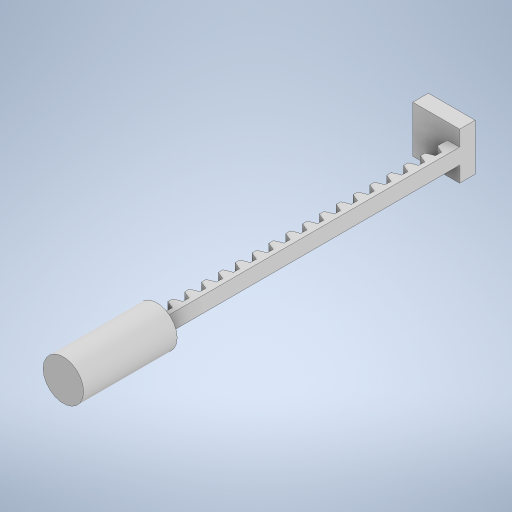
# Autodesk Inventor part: Lineartranslator
Saved by Autodesk Inventor 2024 (Build 280153000, 153)
## iProperties
Created: 2024-01-09
Part Number: Lineartranslator
Material: Generisch
Document SubType Name: Modeling
Designer: mariu
Density: 1 g/cm^3
Appearance: Vorgabe
Author: mariu
Autodesk Inventor part; units mm, degrees
ref_plane "YZ Plane" through (0, 0, 0) normal (1, 0, 0) x (0, 1, 0)
ref_plane "XZ Plane" through (0, 0, 0) normal (0, 1, 0) x (-1, 0, 0)
ref_plane "XY Plane" through (0, 0, 0) normal (0, 0, 1) x (1, 0, 0)
sketch "Skizze2" plane through (0, 0, 0) normal (0, 0, 1) x (1, 0, 0)
  circle A0 centre (0, 0) radius 12.5 construction
  circle A1 centre (0, 0) radius 15
  line L0 (-15, 0) -> (-12.5, 0)
  arc A2 (-12.4599, -1) -> (-14.8661, -2) centre (-8.8919, -12.9799) ccw
  arc A3 (-14.8661, 2) -> (-12.4599, 1) centre (-8.8919, 12.9799) ccw
  arc A4 (-14.8661, 2) -> (-14.8661, -2) centre (0, 0) ccw
  arc A5 (-12.4599, 1) -> (-12.4599, -1) centre (0, 0) ccw
  circle A6 centre (0, 0) radius 15
  line L1 (-12.4599, 1) -> (-12.4599, -1)
  line L2 (-12.4599, 1) -> (-12.4599, 21)
  line L3 (-12.4599, -1) -> (-12.4599, -21)
  line L4 (-14.8661, -2) -> (-14.8661, -21)
  line L5 (-12.4599, -21) -> (-14.8661, -21)
  line L6 (-14.8661, 2) -> (-14.8661, 21)
  line L7 (-14.8661, 21) -> (-12.4599, 21)
  line L8 (-12.4599, 21) -> (-10.9599, 21)
  line L9 (-10.9599, 21) -> (-10.9599, -21)
  line L10 (-10.9599, -21) -> (-12.4599, -21)
  line L11 (-14.8661, 2) -> (-14.8661, 2.9)
  line L12 (-14.8661, 2.9) -> (-12.4599, 2.9)
  line L13 (-14.8661, -2) -> (-14.8661, -2.9)
  line L14 (-14.8661, -2.9) -> (-12.4599, -2.9)
  point P0 (-13.75, 0)
  point P1 (-15, 0)
  point P2 (-12.4599, -8.3516)
  point P3 (-10.9599, -10.2411)
  point P4 (-10.9599, 10.2411)
  point P5 (-12.4599, 8.3516)
  dimension "d5" = 25
  dimension "d6" = 12.5
  dimension "d7" = 4
  dimension "d8" = 2
  dimension "d9" = 13.75
  dimension "d11" = 30
  dimension "d12" = 20
  dimension "d13" = 20
  dimension "d14" = 1.5
  dimension "d17" = 0.9
  dimension "d18" = 0.9
  constraints: 30 end point, 15 point on circle, 7 centre point, 7 coincident, 6 perpendicular, 6 point on line, 3 horizontal, 2 concentric, 2 vertical, 1 horizontal alignment, 1 midpoint, 1 other
  measures "d5" diameter of A0
  measures "d6" radius of A2
  measures "d7" distance of L6.start L4.start
  measures "d8" distance of L1.start L1.end
  measures "d9" distance of point (0, 0) point (-13.75, 0)
  measures "d11" diameter of A6
  measures "d12" distance of L1.start L2.end
  measures "d13" distance of L1.end L3.end
  measures "d14" distance of L2.end L8.end
  measures "d17" distance of L6.start L11.end
  measures "d18" distance of L4.start L13.end
extrude "Extrusion1" add sketch "Skizze2" along normal blind 5 contours L6 L12 A1 | A1 L12 L2 A3 | L2 A1 L9 L3 L1 | A2 L3 L14 A1 | A1 L14 L4
pattern_linear "Rechteckige Anordnung1" count 20 spacing 5.4 along (0, 1, 0) of "Extrusion1"
sketch "Skizze3" plane through (-12.4599, 105.5, 0) normal (-1, 0, 0) x (0, 0, 1)
  line L0 (5, -115.7411) -> (5, 7.3411) projected
  line L1 (5, 2.3411) -> (0, 2.3411)
  line L2 (0, -115.7411) -> (0, 7.3411) projected
  line L3 (0, 2.3411) -> (0, 7.3411)
  line L4 (0, 7.3411) -> (5, 7.3411)
  line L5 (5, 7.3411) -> (5, 2.3411)
  point P0 (0, -105.5)
  point P1 (2.5, 7.3411)
  dimension "d22" = 5
  constraints: 8 end point, 3 perpendicular, 1 horizontal, 1 midpoint, 1 point on line
  measures "d22" distance from line of point (2.5, 7.341) L1
extrude "Extrusion2" cut sketch "Skizze3" against normal blind 5
sketch "Skizze4" plane through (-12.4599, 107.8411, 5) normal (0, 1, 0) x (1, 0, 0)
  line L0 (1.5, 5) -> (1.5, 0) projected
  line L1 (1.5, 0) -> (1.5, 5)
  line L2 (1.5, 5) -> (1.5, 10)
  line L3 (1.5, 10) -> (-13.5, 10)
  line L4 (1.5, 2.5) -> (-2.4061, 2.5) construction
  line L5 (-2.4061, 5) -> (-2.4061, 0) projected
  line L6 (-13.5, 10) -> (-13.5, 5)
  line L7 (1.5, 0) -> (1.5, 5)
  line L8 (1.5, 0) -> (1.5, -5)
  line L9 (1.5, -5) -> (-13.5, -5)
  line L10 (-13.5, -5) -> (-13.5, 5)
  point P0 (12.4599, 5)
  dimension "d25" = 5
  dimension "d26" = 15
  constraints: 18 end point, 4 symmetric about line, 2 midpoint, 1 collinear, 1 horizontal, 1 point on line, 1 vertical
  measures "d25" distance of L0.start L2.end
  measures "d26" distance of L2.end L3.end
extrude "Extrusion3" add sketch "Skizze4" along normal blind 5
sketch "Skizze5" plane through (0, 0, 5) normal (0, 0, 1) x (1, 0, 0)
  line L0 (-14.8661, 105.5) -> (-14.8661, 104.6) projected
  line L1 (-12.4599, 107.8411) -> (-10.9599, 107.8411) projected
  line L2 (-14.8661, 105.5) -> (-12.4599, 105.5)
  line L3 (-12.4599, 105.5) -> (-12.4599, 107.8411)
  line L4 (-12.4599, 107.8411) -> (-14.8661, 107.8411)
  line L5 (-14.8661, 107.8411) -> (-14.8661, 105.5)
  point P0 (0, 0)
  constraints: 8 end point, 2 parallel, 1 horizontal, 1 perpendicular
extrude "Extrusion4" add sketch "Skizze5" against normal blind 5
sketch "Skizze7" plane through (-12.4599, -8.3516, 0) normal (-1, 0, 0) x (0, 0, 1)
  line L0 (5, -1.8894) -> (5, 116.1927) projected
  line L1 (0, -1.8894) -> (5, -1.8894) projected
  line L2 (5, 2.1106) -> (0, 2.1106)
  line L3 (0, 2.1106) -> (0, -1.8894)
  line L4 (0, -1.8894) -> (5, -1.8894)
  line L5 (5, -1.8894) -> (5, 2.1106)
  point P0 (0, 8.3516)
  dimension "d34" = 4
  constraints: 8 end point, 2 parallel, 1 horizontal, 1 perpendicular, 1 point on line
  measures "d34" distance between parallel lines of L1 L2
extrude "Extrusion6" cut sketch "Skizze7" against normal blind 10
sketch "Skizze8" plane through (-14.8661, -2.9, 0) normal (0, -1, 0) x (1, 0, 0)
  circle A0 centre (2.57, 2.5) radius 6.5
  line L0 (0, 0) -> (0, 5) projected
  line L1 (0, 5) -> (2.4061, 5) projected
  point P0 (14.8661, 0)
  dimension "d37" = 13
  dimension "d38" = 2.57
  dimension "d39" = 2.5
  constraints: 1 centre point
  measures "d37" diameter of A0
  measures "d38" distance from line of L0 A0.centre
  measures "d39" distance from line of A0.centre L1
extrude "Extrusion7" add sketch "Skizze8" along normal mid plane 30
